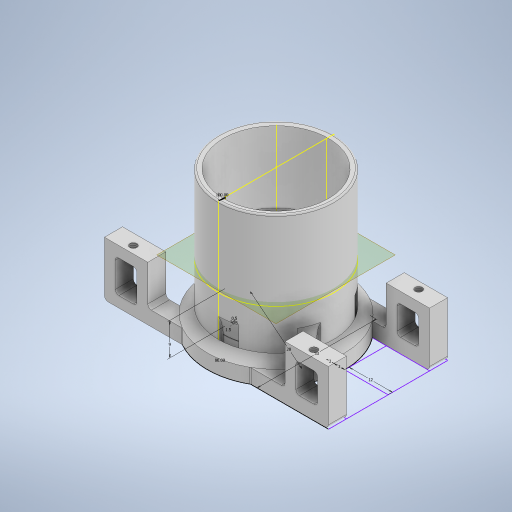
# Autodesk Inventor part: 다단로켓벨브1
Saved by Autodesk Inventor 2023 (Build 270158000, 158)
## iProperties
Created: 2023-08-24
Part Number: 다단로켓벨브1
Material: 일반
Document SubType Name: Modeling
Designer: rlatk
Density: 1 g/cm^3
Appearance: 기본값
Author: rlatk
Autodesk Inventor part; units mm, degrees
ref_plane "YZ Plane" through (0, 0, 0) normal (1, 0, 0) x (0, 1, 0)
ref_plane "XZ Plane" through (0, 0, 0) normal (0, 1, 0) x (-1, 0, 0)
ref_plane "XY Plane" through (0, 0, 0) normal (0, 0, 1) x (1, 0, 0)
sketch "스케치1" plane through (0, 0, 0) normal (0, 1, 0) x (-1, 0, 0)
  circle A0 centre (0, 0) radius 14
  circle A1 centre (0, 0) radius 16
  circle A2 centre (0, 0) radius 19
  line L0 (-9.4207, 16.5) -> (-9.4207, -16.5)
  line L1 (-19, 0) -> (-31, 0)
  line L2 (-9.4207, 16.5) -> (-31, 16.5)
  line L3 (-31, 11.5) -> (-9.4207, 11.5)
  line L4 (-9.4207, 11.5) -> (-9.4207, 16.5)
  line L5 (-9.4207, -16.5) -> (-31, -16.5)
  line L6 (-31, -11.5) -> (-9.4207, -11.5)
  line L7 (-31, 0) -> (-31, 16.5)
  line L8 (-31, 0) -> (-31, -16.5)
  line L9 (-19, -16.5) -> (-19, 16.5)
  point P0 (-15.1245, -11.5)
  point P1 (-15.1245, 11.5)
  point P2 (-9.4207, -11.5)
  point P3 (-9.4207, 11.5)
  point P4 (-19, 11.5)
  point P5 (-19, -11.5)
  dimension "d0" = 28
  dimension "d1" = 2
  dimension "d26" = 3
  dimension "d51" = 33
  dimension "d53" = 12
  constraints: 20 end point, 5 point on line, 3 centre point, 3 point on circle, 2 horizontal, 2 perpendicular, 1 coincident, 1 parallel, 1 symmetric about line, 1 vertical
  measures "d0" diameter of A0
  measures "d1" radial gap between concentric circles of A0 A1
  measures "d26" radial gap between concentric circles of A1 A2
  measures "d51" distance of L0.start L0.end
  measures "d53" distance of L1.start L1.end
extrude "돌출1" add sketch "스케치1" along normal blind 39 contours A0 L0 A1 | A0 L0 L6 A1 L3 | L3 A1 L0 | L0 A1 L6
sketch "스케치2" plane through (0, 0, 0) normal (0, 1, 0) x (-1, 0, 0)
  point P0 (0, 0)
ref_plane "작업 평면1" through (0, 18, 0) normal (0, -1, 0) x (1, 0, 0)
sketch "스케치3" plane through (0, 39, 0) normal (0, 1, 0) x (1, 0, 0)
  point P0 (0, 0)
sketch "스케치4" plane through (0, 18, 0) normal (0, -1, 0) x (1, 0, 0)
  circle A0 centre (0, 0) radius 14 projected
  circle A1 centre (0, 0) radius 14
  circle A2 centre (0, 0) radius 3.85
  dimension "d5" = 7.7
  constraints: 2 centre point, 2 coincident, 1 concentric
  measures "d5" diameter of A2
extrude "돌출2" add sketch "스케치4" along normal blind 1 and the other way blind 1
sketch "스케치5" plane through (0, 0, 0) normal (1, 0, 0) x (0, 1, 0)
  line L0 (17, 14) -> (0, 14) projected
  line L1 (0, 14) -> (0, -14) projected
  line L2 (17, -14) -> (17, 14) projected
  line L3 (17, -14) -> (0, -14) projected
  line L4 (8.75, 14) -> (7.25, 14)
  line L5 (7.25, 14) -> (7.25, 12.5)
  line L6 (7.25, 12.5) -> (8.75, 12.5)
  line L7 (8.75, 12.5) -> (8.75, 14)
  line L8 (8.75, 14) -> (8.25, 12.5)
  line L9 (7.25, 13.9506) -> (7.75, 12.5)
  line L10 (0, 16) -> (39, 16) projected
  line L11 (0, -16) -> (0, 16) projected
  line L12 (0, -16) -> (39, -16) projected
  line L13 (0, 16) -> (0.3527, 14)
  line L14 (17, 14) -> (0, 14) projected
  line L15 (0, 16) -> (2.0309, 16) construction
  line L16 (0, 16) -> (0, 14)
  line L17 (0.3527, 14) -> (0, 14)
  line L18 (-8.2062, 0) -> (49.237, 0) projected
  line L19 (39, -16) -> (39, 16) projected
  line L20 (39, -16) -> (39, 16) projected
  line L21 (0, -16) -> (0, 16) projected
  line L22 (39, 14) -> (19, 14) projected
  line L23 (39, -14) -> (19, -14) projected
  line L24 (39, 16) -> (39, 14)
  line L25 (39, 16) -> (38.6473, 14)
  line L26 (39, 14) -> (19, 14) projected
  line L27 (39, 16) -> (41.0309, 16) construction
  line L28 (38.6473, 14) -> (39, 14)
  line L29 (39, 13) -> (19, 13) projected
  point P0 (0, 0)
  point P1 (8.75, 13.25)
  point P2 (8, 14)
  dimension "d10" = 1.5
  dimension "d11" = 1.5
  dimension "d13" = 9
  dimension "d14" = 0.5
  dimension "d15" = 0.5
  dimension "d24" = 80
  dimension "d32" = 100
  constraints: 28 end point, 6 point on line, 4 horizontal, 3 collinear, 2 equal length, 2 midpoint, 2 parallel, 1 perpendicular, 1 other
  measures "d10" distance of L6.end L5.end
  measures "d11" distance of L5.end L4.end
  measures "d13" distance from line of L2 point (8, 14)
  measures "d14" distance of L8.end L6.end
  measures "d15" distance of L5.end L9.end
  measures "d24" angle of L13 L15
  measures "d32" angle of L25 L27
coil "코일1" sketch "스케치5" operation add axis through (0, -10, 0) along (0, 1, 0) pitch 3 turns 2 hand right contours L8 L6 L9 L5 L0
revolve "회전1" cut sketch "스케치5" angle 360 about axis through (0, -10, 0) along (0, 1, 0) contours L0 L11 L13
extrude "돌출3" add sketch "스케치1" along normal blind 4 contours L0 A2 A1 | A1 L3 A2 L0 | A1 L6 A2 L3 | L0 A2 L6 A1
sketch "스케치6" plane through (0, 0, 0) normal (1, 0, 0) x (0, 1, 0)
  line L0 (4, -19) -> (4, 19) projected
  line L1 (4, 19) -> (5.7321, 16)
  line L2 (4, 16) -> (39, 16) projected
  line L3 (4, 19) -> (7.4641, 19) construction
  line L4 (5.7321, 16) -> (4, 16)
  line L5 (4, 16) -> (4, 19)
  line L6 (-7.8, 0) -> (46.8, 0) projected
  point P0 (0, 0)
  dimension "d29" = 60
  constraints: 8 end point, 2 point on line, 1 equal length, 1 horizontal, 1 perpendicular
  measures "d29" angle of L1 L3
revolve "회전2" add sketch "스케치6" angle 360 about axis through (0, -10, 0) along (0, 1, 0)
revolve "회전3" cut sketch "스케치5" angle 360 about axis through (0, -10, 0) along (0, 1, 0) contours L22 L25 L19
fillet "모깎기2" radius 0.4 2 edges at (11.3137, 39, -11.3137) (-11.3137, 39, 11.3137)
sketch "스케치7" plane through (0, 0, 0) normal (1, 0, 0) x (0, 1, 0)
  line L0 (6.3094, 16) -> (6.3094, -16) projected
  line L1 (6.3094, 16) -> (11.3094, 16)
  line L2 (5.7321, 16) -> (38.5233, 16) projected
  line L3 (11.3094, 16) -> (6.1446, 14.6071)
  line L4 (6.1446, 14.6071) -> (2.1446, 14.6071)
  line L5 (2.1446, 14.6071) -> (0, 16)
  line L6 (0, 16) -> (0.3527, 14) projected
  line L7 (6.3094, 16) -> (2.3094, 16)
  line L8 (2.3094, 16) -> (0, 17.5)
  line L9 (0, -18) -> (0, 18) projected
  arc A0 (6.1446, 14.6071) -> (11.3094, 16) centre (6.2179, 24.6068) ccw
  arc A1 (0, 16) -> (2.1446, 14.6071) centre (3.1368, 18.482) ccw
  arc A2 (0, 17.5) -> (2.3094, 16) centre (3.2004, 19.8995) ccw
  line L10 (-7.9598, 0) -> (46.8266, 0) projected
  point P0 (0, 0)
  point P1 (6.3094, 14.6515)
  point P2 (6.3094, 14.6072)
  dimension "d35" = 5
  dimension "d36" = 4
  dimension "d37" = 1.5
  dimension "d38" = 10
  dimension "d39" = 4
  dimension "d40" = 4
  constraints: 12 end point, 6 point on circle, 5 point on line, 3 centre point, 2 parallel, 1 other
  measures "d35" distance of L1.start L1.end
  measures "d36" distance of L3.end L4.end
  measures "d37" distance of L8.end L5.end
  measures "d38" radius of A0
  measures "d39" radius of A1
  measures "d40" radius of A2
revolve "회전4" cut sketch "스케치7" angle 18 about axis through (0, -10, 0) along (0, 1, 0) picked at (9.1173, 15.2988) contours L1 L3 L0 | L0 L3 L4 L5 L9 A2 L7 L2 | L3 A0 L0 | A1 L5
pattern_circular "원형 패턴1" count 6 over 360 about axis through (0, -10, 0) along (0, 1, 0) of "회전4"
fillet "모깎기3" radius 1 1 edges at (14, 17, 0)
sketch "스케치8" plane through (0, 17, 0) normal (0, -1, 0) x (1, 0, 0)
  circle A0 centre (0, 0) radius 16 projected
  circle A1 centre (0, 0) radius 15.5305 projected
sketch "스케치9" plane through (0, 19, 0) normal (0, 1, 0) x (1, 0, 0)
  circle A0 centre (0, 0) radius 14.5
  circle A1 centre (0, 0) radius 14
  dimension "d46" = 29
  dimension "d47" = 28
  constraints: 2 centre point, 2 coincident
  measures "d46" diameter of A0
  measures "d47" diameter of A1
extrude "돌출4" cut sketch "스케치9" along normal blind 39 contours A0 | A1
extrude "돌출6" add sketch "스케치1" along normal blind 4 contours A2 L3 L9 L2 | L5 L9 L6 A2 | L9 L3 L7 L2 | L5 L8 L6 L9
extrude "돌출7" add sketch "스케치1" along normal blind 15 contours L9 L3 L7 L2 | L5 L8 L6 L9
sketch "스케치10" plane through (31, 0, -16.5) normal (0, 0, -1) x (-1, 0, 0)
  line L0 (0, 0) -> (21.5793, 0) projected
  line L1 (21.5793, 4) -> (21.5793, 0) projected
  line L2 (12, 4) -> (21.5793, 4) projected
  line L3 (12, 4) -> (12, 15) projected
  line L4 (0, 15) -> (12, 15) projected
  line L5 (0, 0) -> (0, 15) projected
  line L6 (12, 4) -> (12, 15) projected
  line L7 (12, 4) -> (3, 4)
  line L8 (3, 4) -> (3, 12)
  line L9 (3, 12) -> (12, 12)
  line L10 (12, 12) -> (12, 4)
  point P0 (31, 0)
  point P1 (12, 12)
  dimension "d61" = 3
  dimension "d62" = 3
  constraints: 8 end point, 2 parallel, 1 horizontal, 1 perpendicular
  measures "d61" distance between parallel lines of L4 L9
  measures "d62" distance between parallel lines of L5 L8
extrude "돌출8" cut sketch "스케치10" against normal blind 33 contours L7 L8 L9 L3
sketch "스케치11" plane through (0, 15, 0) normal (0, 1, 0) x (1, 0, 0)
  line L0 (31, 16.5) -> (19, 16.5) projected
  line L1 (19, 16.5) -> (19, 11.5) projected
  line L2 (19, -16.5) -> (31, -16.5) projected
  line L3 (19, -11.5) -> (19, -16.5) projected
  point P0 (0, 0)
  point P1 (25, 14.5)
  point P2 (25, -14.5)
  dimension "d65" = 2
  dimension "d66" = 6
  dimension "d67" = 2
  dimension "d68" = 6
  measures "d65" distance from line of L0 point (25, 14.5)
  measures "d66" distance from line of L1 point (25, 14.5)
  measures "d67" distance from line of L2 point (25, -14.5)
  measures "d68" distance from line of L3 point (25, -14.5)
hole "구멍1" at (25, 15, 14.5) at (25, 15, -14.5) direction (0, -1, 0) diameter 2.013 depth 7.6 tip angle 118 thread size "M2.5x0.45" class "6H" standard "ISO Metric profile"
sketch "스케치12" plane through (19, 12, -16.5) normal (0, -1, 0) x (1, 0, 0)
  line L0 (-3.8755, 5) -> (12, 5) projected
  line L1 (12, 0) -> (-9.5793, 0) projected
  line L2 (12, 5) -> (12, 0) projected
  line L3 (0, 0) -> (0, 5) projected
  line L4 (9, 0) -> (0, 0) projected
  line L5 (0, 5) -> (3, 5)
  line L6 (3, 5) -> (3, 0)
  line L7 (3, 0) -> (0, 0)
  line L8 (0, 0) -> (0, 5)
  line L9 (-9.5793, 33) -> (12, 33) projected
  arc A0 (-9.5793, 33) -> (-9.5793, 0) centre (-19, 16.5) ccw projected
  arc A1 (-3.8755, 5) -> (-3.8755, 28) centre (-19, 16.5) ccw projected
  line L10 (12, 28) -> (-3.8755, 28) projected
  line L11 (12, 33) -> (12, 28) projected
  point P0 (3, 0)
  point P1 (3, 5)
  dimension "d76" = 3
  constraints: 8 end point, 2 parallel, 1 horizontal, 1 perpendicular, 1 point on line
  measures "d76" distance of L6.end L7.end
extrude "돌출9" add sketch "스케치12" along normal blind 12 contours L0 L6 L1 L3
sketch "스케치13" plane through (0, 15, 0) normal (0, 1, 0) x (1, 0, 0)
  circle A0 centre (25, -14.5) radius 1.0065 projected
  line L0 (19, -16.5) -> (31, -16.5) projected
  line L1 (31, -16.5) -> (31, -11.5) projected
  line L2 (31, -11.5) -> (19, -11.5) projected
  line L3 (19, -11.5) -> (19, -16.5) projected
  line L4 (28, -11.5) -> (19, -11.5) projected
  line L5 (19, -16.5) -> (22, -16.5)
  line L6 (22, -16.5) -> (22, -11.5)
  line L7 (22, -11.5) -> (19, -11.5)
  line L8 (19, -11.5) -> (19, -16.5)
  point P0 (0, 0)
  point P1 (22, -11.5)
  dimension "d79" = 3
  constraints: 8 end point, 2 parallel, 1 horizontal, 1 perpendicular, 1 point on line
  measures "d79" distance of L7.end L6.end
extrude "돌출10" add sketch "스케치13" against normal blind 12 contours L3 L2 L6 L0
mirror "미러1" about plane through (0, 0, 0) normal (1, 0, 0) of "돌출7", "돌출6"
mirror "미러2" about plane through (0, 0, 0) normal (1, 0, 0) of "구멍1"
sketch "스케치14" plane through (-31, 15, 16.5) normal (0, 0, 1) x (1, 0, 0)
  point P0 (31, -15)
sketch "스케치15" plane through (-31, 15, 16.5) normal (0, 0, 1) x (1, 0, 0)
  line L0 (21.5793, -15) -> (0, -15) projected
  line L1 (21.5793, -11) -> (21.5793, -15) projected
  line L2 (21.5793, -11) -> (12, -11) projected
  line L3 (12, -11) -> (12, 0) projected
  line L4 (12, 0) -> (0, 0) projected
  line L5 (0, -15) -> (0, 0) projected
  line L6 (3, -3) -> (9, -3)
  line L7 (9, -3) -> (9, -12)
  line L8 (9, -12) -> (3, -12)
  line L9 (3, -12) -> (3, -3)
  point P0 (31, -15)
  point P1 (3, -7.5)
  dimension "d83" = 3
  dimension "d84" = 3
  dimension "d85" = 3
  dimension "d86" = 3
  constraints: 8 end point, 2 parallel, 1 horizontal, 1 midpoint, 1 perpendicular
  measures "d83" distance between parallel lines of L4 L6
  measures "d84" distance between parallel lines of L0 L8
  measures "d85" distance between parallel lines of L7 L3
  measures "d86" distance from line of L5 point (3, -7.5)
extrude "돌출11" cut sketch "스케치15" against normal blind 33 contours L6 L7 L8 L9
fillet "모깎기6" radius 1 28 edges at (9.4207, 2, -16.5) (-9.4207, 2, -16.5) (22, 12, -14) (28, 12, -14) (22, 4, -14) (28, 4, -14) (-22, 3, -14) (-28, 3, -14) (-22, 12, -14) (-28, 12, -14) (19, 4, -14) (-19, 4, -14) (31, 0, -14) (31, 0, 14) (-31, 0, -14) (22, 12, 14) (28, 12, 14) (22, 4, 14) (28, 4, 14) (9.4207, 2, 16.5) (19, 4, 14) (-19, 4, 14) (-28, 3, 14) (-22, 3, 14) (-28, 12, 14) (-22, 12, 14) (-31, 0, 14) (-9.4207, 2, 16.5)
